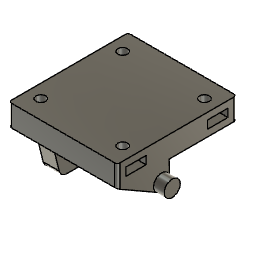
Camera Mount Rev2 (Autodesk Fusion 360 design; units mm, degrees)
Autodesk Fusion 360 part; units mm, degrees
note: some values were not read from the file. Chosen so that the rebuilt part matches the saved one: which face or edge a step refers to. Set by a fixed rule: which sketch regions a step uses.
sketch "Sketch1" plane through (0, 0, 0) normal (0, 0, 1) x (1, 0, 0)
  line L0 (-40.6439, 21.225) -> (-81.2739, 21.225)
  line L1 (-81.2739, 21.225) -> (-81.2739, -23.405)
  line L2 (-81.2739, -23.405) -> (-40.6439, -23.405)
  line L3 (-40.6439, -23.405) -> (-40.6439, 21.225)
  circle A0 centre (-76.2739, 14.225) radius 1.8
  circle A1 centre (-76.2739, -16.405) radius 1.8
  circle A2 centre (-45.6439, -16.405) radius 1.8
  circle A3 centre (-45.6439, 14.225) radius 1.8
  line L4 (-72.4989, 18) -> (-80.0489, 18)
  line L5 (-80.0489, 18) -> (-80.0489, 10.45)
  line L6 (-80.0489, 10.45) -> (-72.4989, 10.45)
  line L7 (-72.4989, 10.45) -> (-72.4989, 18)
  line L8 (-72.4989, 18) -> (-80.0489, 10.45) construction
  line L9 (-80.0489, 18) -> (-72.4989, 10.45) construction
  line L10 (-80.0489, 18) -> (-81.2739, 18)
  line L11 (-80.0489, 10.45) -> (-81.2739, 10.45)
  line L12 (-79.405, 17) -> (-80.63, 17)
  line L13 (-79.405, 9.45) -> (-80.63, 9.45)
  line L14 (-72.4989, -12.63) -> (-80.0489, -12.63)
  line L15 (-80.0489, -12.63) -> (-80.0489, -20.18)
  line L16 (-80.0489, -20.18) -> (-72.4989, -20.18)
  line L17 (-72.4989, -20.18) -> (-72.4989, -12.63)
  line L18 (-72.4989, -12.63) -> (-80.0489, -20.18) construction
  line L19 (-80.0489, -12.63) -> (-72.4989, -20.18) construction
  line L20 (-49.4189, -12.63) -> (-41.8689, -12.63)
  line L21 (-41.8689, -12.63) -> (-41.8689, -20.18)
  line L22 (-41.8689, -20.18) -> (-49.4189, -20.18)
  line L23 (-49.4189, -20.18) -> (-49.4189, -12.63)
  line L24 (-49.4189, -12.63) -> (-41.8689, -20.18) construction
  line L25 (-41.8689, -12.63) -> (-49.4189, -20.18) construction
  line L26 (-49.4189, 18) -> (-41.8689, 18)
  line L27 (-41.8689, 18) -> (-41.8689, 10.45)
  line L28 (-41.8689, 10.45) -> (-49.4189, 10.45)
  line L29 (-49.4189, 10.45) -> (-49.4189, 18)
  line L30 (-49.4189, 18) -> (-41.8689, 10.45) construction
  line L31 (-41.8689, 18) -> (-49.4189, 10.45) construction
  line L32 (-41.8689, 18) -> (-40.6439, 18)
  line L33 (-41.8689, 10.45) -> (-40.6439, 10.45)
  line L34 (-41.8689, -12.63) -> (-40.6439, -12.63)
  line L35 (-41.8689, -20.18) -> (-40.6439, -20.18)
  line L36 (-80.0489, -12.63) -> (-81.2739, -12.63)
  line L37 (-80.0489, -20.18) -> (-81.2739, -20.18)
  line L38 (-70.0739, 21.225) -> (-64.0739, 21.225)
  line L39 (-64.0739, 21.225) -> (-64.0739, -23.405)
  line L40 (-64.0739, -23.405) -> (-70.0739, -23.405)
  line L41 (-70.0739, -23.405) -> (-70.0739, 21.225)
  point P0 (-76.2739, 14.225)
  point P1 (-76.2739, -16.405)
  point P2 (-45.6439, -16.405)
  point P3 (-45.6439, 14.225)
  dimension "d80" = 44.63
  dimension "d81" = 40.63
  dimension "d82" = 3.6
  dimension "d83" = 7
  dimension "d84" = 5
  dimension "d85" = 3.6
  dimension "d86" = 3.6
  dimension "d87" = 3.6
  dimension "d88" = 5
  dimension "d89" = 7
  dimension "d90" = 5
  dimension "d91" = 7
  dimension "d92" = 5
  dimension "d93" = 7
  dimension "d94" = 7.55
  dimension "d95" = 7.55
  dimension "d96" = 7.55
  dimension "d97" = 7.55
  dimension "d98" = 7.55
  dimension "d99" = 7.55
  dimension "d100" = 7.55
  dimension "d101" = 7.55
  dimension "d102" = 6
  dimension "d103" = 11.2
  constraint horizontal L0
  constraint vertical L1
  constraint horizontal L2
  constraint vertical L3
  constraint horizontal L4
  constraint perpendicular L4 L5
  constraint parallel L4 L6
  constraint parallel L5 L7
  constraint coincident L8 P0
  constraint coincident L9 P0
  constraint coincident P0 A0.centre
  constraint coincident L1 L10.end
  constraint perpendicular L1 L10
  constraint coincident L1 L11.end
  constraint perpendicular L1 L11
  constraint horizontal L14
  constraint perpendicular L14 L15
  constraint parallel L14 L16
  constraint parallel L15 L17
  constraint coincident L18 P1
  constraint coincident L19 P1
  constraint coincident P1 A1.centre
  constraint horizontal L20
  constraint perpendicular L20 L21
  constraint parallel L20 L22
  constraint parallel L21 L23
  constraint coincident L24 P2
  constraint coincident L25 P2
  constraint coincident P2 A2.centre
  constraint horizontal L26
  constraint perpendicular L26 L27
  constraint parallel L26 L28
  constraint parallel L27 L29
  constraint coincident L30 P3
  constraint coincident L31 P3
  constraint coincident P3 A3.centre
  constraint coincident L3 L32.end
  constraint perpendicular L3 L32
  constraint coincident L3 L33.end
  constraint perpendicular L3 L33
  constraint coincident L3 L34.end
  constraint perpendicular L3 L34
  constraint coincident L3 L35.end
  constraint perpendicular L3 L35
  constraint coincident L1 L36.end
  constraint perpendicular L1 L36
  constraint coincident L1 L37.end
  constraint perpendicular L1 L37
  constraint horizontal L38
  constraint vertical L39
  constraint horizontal L40
  constraint vertical L41
  constraint coincident L0 L38.start
  measures "d80" distance of L0.end L1.end
  measures "d81" distance of L0.start L0.end
  measures "d82" diameter of A0
  measures "d83" distance of L0 P0
  measures "d84" distance of L1 P0
  measures "d85" diameter of A1
  measures "d86" diameter of A2
  measures "d87" diameter of A3
  measures "d88" distance of L3 P3
  measures "d89" distance of L0 P3
  measures "d90" distance of L3 P2
  measures "d91" distance of L2 P2
  measures "d92" distance of L1 P1
  measures "d93" distance of L2 P1
  measures "d94" distance of L5.end L6.end
  measures "d95" distance of L4.start L6.end
  measures "d96" distance of L14.start L16.end
  measures "d97" distance of L14.start L14.end
  measures "d98" distance of L21.end L22.end
  measures "d99" distance of L20.start L22.end
  measures "d100" distance of L27.end L28.end
  measures "d101" distance of L26.start L28.end
  measures "d102" distance of L38.start L38.end
  measures "d103" distance of L1 L41
extrude "Extrude16" add sketch "Sketch1" along normal blind 8
extrude "Extrude17" cut sketch "Sketch1" along normal blind 3 from surface at 2.5 contours L3 L27 L32 L33 | L26 L27 L28 L29 | L3 L21 L34 L35 | L1 L5 L10 L11 | L20 L21 L22 L23 | L4 L5 L6 L7 | L1 L15 L36 L37 | L14 L15 L16 L17
extrude "Extrude18" add sketch "Sketch1" against normal blind 12.1 contours L0 L2 L38 L39 L40 L41
sketch "Sketch7" plane through (-70.0739, 0, 0) normal (-1, 0, 0) x (0, -1, 0)
  line L0 (23.405, 0) -> (-21.225, 0)
  line L1 (-21.225, 0) -> (-21.225, -12.1)
  line L2 (-21.225, -12.1) -> (23.405, -12.1)
  line L3 (23.405, -12.1) -> (23.405, 0)
  line L4 (23.405, -6.05) -> (-21.225, -6.05)
  line L5 (12.59, -12.1) -> (-10.41, -12.1)
  line L6 (-10.41, -12.1) -> (-10.41, 0)
  line L7 (-10.41, 0) -> (12.59, 0)
  line L8 (12.59, 0) -> (12.59, -12.1)
  line L9 (12.59, -12.1) -> (-10.41, 0) construction
  line L10 (-10.41, -12.1) -> (12.59, 0) construction
  circle A0 centre (-13.41, -6.05) radius 0.5
  circle A1 centre (15.59, -6.05) radius 0.5
  line L11 (23.405, 0) -> (20.405, -12.1)
  line L12 (-21.225, 0) -> (-18.225, -12.1)
  circle A2 centre (6.84, -6.05) radius 2.5
  circle A3 centre (6.84, -6.05) radius 3
  line L13 (23.405, 0) -> (8.3336, -8.6518)
  line L14 (3.84, -6.05) -> (4, 0)
  point P0 (1.09, -6.05)
  dimension "d111" = 23
  dimension "d112" = 1
  dimension "d113" = 14.5
  dimension "d115" = 360
  dimension "d116" = 3
  dimension "d117" = 3
  dimension "d123" = 5
  dimension "d124" = 8.75
  dimension "d125" = 6
  constraint midpoint L3 L4.start
  constraint midpoint L1 L4.end
  constraint horizontal L5
  constraint perpendicular L5 L6
  constraint parallel L5 L7
  constraint parallel L6 L8
  constraint coincident L9 P0
  constraint coincident L10 P0
  constraint midpoint L4 P0
  constraint coincident L4 A0.centre
  constraint coincident L0.start L3.end
  constraint coincident L2 L11.end
  constraint coincident L0.end L1.start
  constraint coincident L2 L12.end
  constraint coincident L4 A2.centre
  constraint concentric A2 A3
  constraint coincident A3 L13.end
  constraint tangent A3 L13
  constraint coincident A3 L14.start
  constraint coincident L4 L14.start
  constraint coincident L7 L14.end
  constraint coincident L0 L14.end
  measures "d111" distance of L6.end L7.end
  measures "d112" diameter of A0
  measures "d113" distance of P0 A0.centre
  measures "d116" distance of L2.end L11.end
  measures "d117" distance of L1.end L12.end
  measures "d123" diameter of A2
  measures "d124" distance of A1.centre A2.centre
  measures "d125" diameter of A3
extrude "Extrude19" cut sketch "Sketch7" against normal up to surface (6 mm away) contours L3 L4 L11 | L4 A2 A3 | L4 A2 A3 | L2 L4 L5 L6 L8 A3 L13 | L0 L4 L7 L8 A3 L14 | L2 L3 L4 L11 | L0 L4 L6 L7 L14 | L4 L8 A3 L13 | L4 A1 | L4 A1 | L1 L4 L12 | L4 A2 | L4 A2 | L1 L2 L4 L12 | L4 A0 | L4 A0
extrude "Extrude20" cut sketch "Sketch1" against normal up to surface (3.1 mm away) from surface at -9 contours L0 L2 L38 L39 L40 L41
extrude "Extrude21" add sketch "Sketch7" against normal blind 2.93 from surface at -26.5 contours L0 L4 L8 L13 | L4 A2 A3 | L4 A2 A3 | L0 L4 L7 L8 A3 L14 | L4 L8 L13 | L4 L8 A3 L13 | L4 A2 | L4 A2
extrude "Extrude22" add sketch "Sketch7" against normal blind 4 from surface at -29.43 contours L4 A2 A3 | L4 A2 A3 | L4 A2 | L4 A2
fillet "Fillet9" radius 3 1 edges at (-67.0739, -21.1736, -9)
fillet "Fillet10" radius 3 1 edges at (-67.0739, 18.9936, -9)
fillet "Fillet11" radius 1 1 edges at (-81.2739, -23.405, 4)
fillet "Fillet12" radius 1 1 edges at (-40.6439, -23.405, 4)
fillet "Fillet13" radius 1 1 edges at (-40.6439, 21.225, 4)
fillet "Fillet14" radius 1 1 edges at (-81.2739, 21.225, 4)
